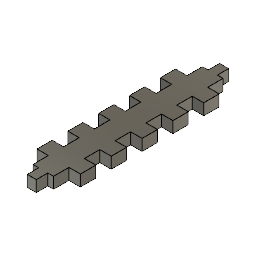
Retrotopside (Autodesk Fusion 360 design; units mm, degrees)
Autodesk Fusion 360 part; units mm, degrees
sketch "Sketch1" plane through (0, 0, 0) normal (0, 0, 1) x (1, 0, 0)
  line L0 (0, 0) -> (9, 0)
  line L1 (9, 0) -> (9, 74)
  line L2 (9, 74) -> (0, 74)
  line L3 (0, 74) -> (0, 0)
  dimension "d5" = 9
  dimension "d6" = 74
  constraint horizontal L0
  constraint vertical L1
  constraint horizontal L2
  constraint vertical L3
  constraint coincident L0.start L3.end
  measures "d5" distance of L0.start L0.end
  measures "d6" distance of L0.start L2.end
extrude "Extrude1" add sketch "Sketch1" along normal blind 5
sketch "Sketch2" plane through (9, 0, 0) normal (1, 0, 0) x (0, 1, 0)
  line L0 (0, 0) -> (74, 0)
  line L1 (74, 0) -> (74, 5)
  line L2 (74, 5) -> (0, 5)
  line L3 (0, 5) -> (0, 0)
  line L4 (6.7273, 5) -> (13.4545, 5)
  line L5 (13.4545, 5) -> (13.4545, 0)
  line L6 (13.4545, 0) -> (6.7273, 0)
  line L7 (6.7273, 0) -> (6.7273, 5)
  line L8 (20.1818, 0) -> (20.1818, 5)
  line L9 (20.1818, 5) -> (26.9091, 5)
  line L10 (26.9091, 5) -> (26.9091, 0)
  line L11 (26.9091, 0) -> (20.1818, 0)
  line L12 (33.6364, 0) -> (33.6364, 5)
  line L13 (33.6364, 5) -> (40.3636, 5)
  line L14 (40.3636, 5) -> (40.3636, 0)
  line L15 (40.3636, 0) -> (33.6364, 0)
  line L16 (47.0909, 0) -> (47.0909, 5)
  line L17 (47.0909, 5) -> (53.8182, 5)
  line L18 (53.8182, 5) -> (53.8182, 0)
  line L19 (53.8182, 0) -> (47.0909, 0)
  line L20 (60.5455, 0) -> (60.5455, 5)
  line L21 (60.5455, 5) -> (67.2727, 5)
  line L22 (67.2727, 5) -> (67.2727, 0)
  line L23 (67.2727, 0) -> (60.5455, 0)
  dimension "d9" = 6.7273
  dimension "d10" = 6.7273
  dimension "d13" = 53.8182
  dimension "d14" = 0
  constraint horizontal L4
  constraint vertical L5
  constraint horizontal L6
  constraint vertical L7
  constraint coincident L0 L5.end
  constraint coincident L2 L4.start
  measures "d9" distance of L4.start L4.end
  measures "d10" distance of L0.start L6.end
extrude "Extrude2" add sketch "Sketch2" along normal blind 5 contours L0 L2 L4 L5 L6 L7 | L0 L2 L8 L9 L10 L11 | L0 L2 L12 L13 L14 L15 | L0 L2 L16 L17 L18 L19 | L0 L2 L20 L21 L22 L23
sketch "Sketch3" plane through (0, 0, 0) normal (-1, 0, 0) x (0, -1, 0)
  line L0 (-74, 0) -> (0, 0)
  line L1 (0, 0) -> (0, 5)
  line L2 (0, 5) -> (-74, 5)
  line L3 (-74, 5) -> (-74, 0)
  line L4 (-67.2727, 5) -> (-60.5455, 5)
  line L5 (-60.5455, 5) -> (-60.5455, 0)
  line L6 (-60.5455, 0) -> (-67.2727, 0)
  line L7 (-67.2727, 0) -> (-67.2727, 5)
  line L8 (-53.8182, 0) -> (-53.8182, 5)
  line L9 (-53.8182, 5) -> (-47.0909, 5)
  line L10 (-47.0909, 5) -> (-47.0909, 0)
  line L11 (-47.0909, 0) -> (-53.8182, 0)
  line L12 (-40.3636, 0) -> (-40.3636, 5)
  line L13 (-40.3636, 5) -> (-33.6364, 5)
  line L14 (-33.6364, 5) -> (-33.6364, 0)
  line L15 (-33.6364, 0) -> (-40.3636, 0)
  line L16 (-26.9091, 0) -> (-26.9091, 5)
  line L17 (-26.9091, 5) -> (-20.1818, 5)
  line L18 (-20.1818, 5) -> (-20.1818, 0)
  line L19 (-20.1818, 0) -> (-26.9091, 0)
  line L20 (-13.4545, 0) -> (-13.4545, 5)
  line L21 (-13.4545, 5) -> (-6.7273, 5)
  line L22 (-6.7273, 5) -> (-6.7273, 0)
  line L23 (-6.7273, 0) -> (-13.4545, 0)
  dimension "d17" = 6.7273
  dimension "d18" = 6.7273
  dimension "d21" = 53.8182
  dimension "d22" = 0
  constraint horizontal L4
  constraint vertical L5
  constraint horizontal L6
  constraint vertical L7
  constraint coincident L0 L5.end
  constraint coincident L2 L4.start
  measures "d17" distance of L4.start L4.end
  measures "d18" distance of L0.start L6.end
extrude "Extrude3" add sketch "Sketch3" along normal blind 5 contours L0 L2 L4 L5 L6 L7 | L0 L2 L8 L9 L10 L11 | L0 L2 L12 L13 L14 L15 | L0 L2 L16 L17 L18 L19 | L0 L2 L20 L21 L22 L23
sketch "Sketch4" plane through (0, 0, 0) normal (0, 0, 1) x (1, 0, 0)
  line L0 (2.5, 0) -> (6.5, 0)
  line L1 (6.5, 0) -> (6.5, -5)
  line L2 (6.5, -5) -> (2.5, -5)
  line L3 (2.5, -5) -> (2.5, 0)
  line L4 (0, 0) -> (9, 0)
  line L5 (6.5, 0) -> (9, 0) construction
  line L6 (0, 0) -> (2.5, 0) construction
  line L7 (2.5, 74) -> (6.5, 74)
  line L8 (6.5, 74) -> (6.5, 79)
  line L9 (6.5, 79) -> (2.5, 79)
  line L10 (2.5, 79) -> (2.5, 74)
  line L11 (9, 74) -> (0, 74)
  line L12 (6.5, 74) -> (9, 74) construction
  line L13 (2.5, 74) -> (0, 74) construction
  dimension "d25" = 5
  dimension "d26" = 4
  dimension "d27" = 4
  dimension "d28" = 5
  constraint horizontal L0
  constraint vertical L1
  constraint horizontal L2
  constraint vertical L3
  constraint coincident L0.start L4
  constraint coincident L4.end L5.end
  constraint coincident L4.start L6.start
  constraint equal L5 L6
  constraint horizontal L7
  constraint vertical L8
  constraint horizontal L9
  constraint vertical L10
  constraint coincident L7.start L11
  constraint coincident L11.start L12.end
  constraint coincident L11.end L13.end
  constraint equal L12 L13
  measures "d25" distance of L0.start L2.end
  measures "d26" distance of L1.end L2.end
  measures "d27" distance of L8.end L9.end
  measures "d28" distance of L7.start L9.end
extrude "Extrude4" add sketch "Sketch4" along normal blind 5
equation "laius = 74 mm"
equation "korgus = 9 mm"
equation "laius_tapp = laius / 11"
equation "paksus = 5 mm"
equation "d5 = korgus"
equation "d6 = laius"
equation "d7 = paksus"
equation "d9 = laius_tapp"
equation "d10 = laius_tapp"
equation "d13 = laius - 3 * laius_tapp"
equation "d15 = paksus"
equation "d17 = laius_tapp"
equation "d18 = laius_tapp"
equation "d21 = laius - 3 * laius_tapp"
equation "d23 = paksus"
equation "d25 = paksus"
equation "d28 = paksus"
equation "d29 = paksus"
